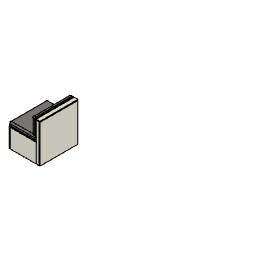
Sofa (Autodesk Fusion 360 design; units mm, degrees)
Autodesk Fusion 360 part; units mm, degrees
sketch "Sketch1" plane through (0, -793.733, 0) normal (0, 1, 0) x (-1, 0, 0)
  line L0 (-1715, -1034) -> (-1715, 1034)
  line L1 (-2315, 1034) -> (-2815, 1034)
  line L2 (-2815, 334) -> (-2315, 334)
  line L3 (-2315, 334) -> (-2315, 1034)
  line L4 (-2315, 1034) -> (-2815, 334) construction
  line L5 (-2815, 1034) -> (-2315, 334) construction
  line L6 (-4545, 1034) -> (-115, 1034)
  line L7 (-2815, 334) -> (-2865, 334)
  line L8 (-2865, 334) -> (-2865, 1034)
  line L9 (-2333, 1016) -> (-2797, 1016)
  line L10 (-2797, 1016) -> (-2797, 352)
  line L11 (-2797, 352) -> (-2333, 352)
  line L12 (-2333, 352) -> (-2333, 1016)
  line L13 (-2333, 1016) -> (-2797, 352) construction
  line L14 (-2797, 1016) -> (-2333, 352) construction
  line L15 (-2865, 334) -> (-2883, 334)
  line L16 (-2883, 334) -> (-2883, 1034)
  line L17 (-2797, 352) -> (-2865, 352)
  line L18 (-2797, 1016) -> (-2865, 1016)
  line L19 (-2815, 1016) -> (-2815, 352)
  line L20 (-2815, 402) -> (-2865, 402)
  line L21 (-2815, 966) -> (-2865, 966)
  line L22 (-2815, 709) -> (-2865, 709)
  line L23 (-2815, 659) -> (-2865, 659)
  line L24 (-2333, 334) -> (-2333, 352)
  line L25 (-2333, 1016) -> (-2333, 1034)
  line L26 (-2815, 1034) -> (-2815, 1016)
  line L27 (-2815, 352) -> (-2815, 334)
  line L28 (-1715, 1034) -> (-3765, 1034)
  line L29 (-3765, 1034) -> (-3765, 0)
  line L30 (-4545, -1034) -> (-1715, -1034)
  line L31 (-3765, 0) -> (-4545, 0)
  line L32 (-4545, 0) -> (-4545, -1034)
  point P0 (-2565, 684)
  point P1 (-2565, 684)
  dimension "d71" = 500
  dimension "d72" = 50
  dimension "d73" = 700
  dimension "d74" = 600
  dimension "d77" = 18
  dimension "d78" = 18
  dimension "d79" = 18
  dimension "d84" = 18
  dimension "d85" = 18
  dimension "d86" = 25
  dimension "d87" = 50
  dimension "d88" = 50
  dimension "d89" = 50
  constraint horizontal L1
  constraint parallel L1 L2
  constraint coincident L4 P1
  constraint coincident L5 P1
  constraint coincident L1.start L6
  constraint horizontal L7
  constraint vertical L8
  constraint coincident L6 L8.end
  constraint horizontal L9
  constraint perpendicular L9 L10
  constraint parallel L9 L11
  constraint parallel L10 L12
  constraint coincident L13 P1
  constraint coincident L14 P1
  constraint coincident P1 P0
  constraint perpendicular L8 L15
  constraint coincident L6 L16.end
  constraint perpendicular L6 L16
  constraint coincident L8 L17.end
  constraint perpendicular L8 L17
  constraint coincident L8 L18.end
  constraint perpendicular L8 L18
  constraint coincident L18 L19.start
  constraint coincident L17 L19.end
  constraint perpendicular L17 L19
  constraint coincident L19 L20.start
  constraint coincident L8 L20.end
  constraint perpendicular L8 L20
  constraint coincident L19 L21.start
  constraint coincident L8 L21.end
  constraint perpendicular L8 L21
  constraint coincident L19 L22.start
  constraint coincident L8 L22.end
  constraint perpendicular L8 L22
  constraint coincident L19 L23.start
  constraint coincident L8 L23.end
  constraint perpendicular L8 L23
  constraint coincident L2 L24.start
  constraint perpendicular L11 L24
  constraint coincident L6 L25.end
  constraint perpendicular L9 L25
  measures "d71" distance of L2.start L2.end
  measures "d72" distance of L2.start L7.end
  measures "d73" distance of L1.start L2.end
  measures "d74" distance of L0 L3
  measures "d77" distance of L3 L12
  measures "d78" distance of L2 L11
  measures "d79" distance of L8 L16
  measures "d84" distance of L10 L19
  measures "d85" distance of L1 L9
  measures "d86" distance of P1 L22
  measures "d87" distance of L22 L23
  measures "d88" distance of L17 L20
  measures "d89" distance of L18 L21
extrude "Extrude1" add sketch "Sketch1" along normal blind 346 contours L1 L2 L3 L6 L12 L24 L25 L28 | L10 L17 L18 L19 makes body 1 at (2315, -678.3997, 567.3333) makes body 2 at (2797, -678.3997, 794.6667)
extrude "Extrude2" add sketch "Sketch1" along normal blind 346 separate body contours L1 L6 L9 L18 L25 L26 L28 | L2 L11 L17 L24 L27 makes body 3 at (2493.6667, -563.0664, 352) makes body 4 at (2493.6667, -563.0664, 1034)
extrude "Extrude3" add sketch "Sketch1" along normal blind 700 separate body contours L6 L8 L18 L26 L28 | L7 L8 L17 L27 makes body 5 at (2831.6667, -327.0664, 334) makes body 6 at (2831.6667, -560.3997, 1016)
extrude "Extrude4" add sketch "Sketch1" along normal blind 700 separate body contours L6 L8 L15 L16 L28 makes body 7
extrude "Extrude1'" add sketch "Sketch1" along normal blind 700 separate body contours L8 L18 L19 L21 | L8 L17 L19 L20 | L8 L19 L22 L23 makes body 8 at (2865, -327.0664, 368.6667) makes body 9 at (2815, -327.0664, 692.3333) makes body 10 at (2815, -327.0664, 999.3333) in component "Wood Support (1)"
extrude "Extrude6" add sketch "Sketch1" along normal blind 18 from surface at 700 separate body contours L6 L8 L18 L26 L28 | L6 L8 L15 L16 L28 | L8 L18 L19 L21 | L7 L8 L17 L27 | L8 L19 L21 L22 | L8 L17 L19 L20 | L8 L19 L22 L23 | L8 L19 L20 L23 makes body 11
extrude "Extrude1''" add sketch "Sketch1" along normal blind 18 from surface at 346 separate body contours L1 L2 L3 L6 L12 L24 L25 L28 | L1 L6 L9 L18 L25 L26 L28 | L9 L10 L11 L12 | L2 L11 L17 L24 L27 | L10 L17 L18 L19 makes body 12 in component "Bottom Pillow"
extrude "Extrude2'" add 1 faces at (2493.6667, -429.733, 692.3333) along direction (0, 1, 0) blind 65 separate body on bodies 12 makes body 13 in component "Bottom Pillow"
extrude "Extrude3'" add 1 faces at (2315, -408.0664, 567.3333) along direction (-1, 0, 0) blind 10 on bodies 13 bodies 13 in component "Bottom Pillow"
extrude "Extrude4'" add 1 faces at (2645, -386.3997, 334) along direction (0, 0, -1) blind 10 on bodies 13 bodies 13 in component "Bottom Pillow"
fillet "Fillet2" radius 25 8 edges at (2305, -397.233, 324) (2815, -397.233, 324) (2560, -364.733, 324) (2815, -364.733, 679) (2815, -397.233, 1034) (2560, -364.733, 1034) (2305, -364.733, 679) (2305, -397.233, 1034) on bodies 13 in component "Bottom Pillow"
fillet "Fillet3" radius 10 8 edges at (2305, -429.733, 679) (2312.3223, -429.733, 1026.6777) (2560, -429.733, 1034) (2807.6777, -429.733, 1026.6777) (2815, -429.733, 679) (2807.6777, -429.733, 331.3223) (2560, -429.733, 324) (2312.3223, -429.733, 331.3223) on bodies 13 in component "Bottom Pillow"
sketch "Sketch1 (2)" plane through (2815, 0, 0) normal (-1, 0, 0) x (0, 0, 1) in component "Back Pillow"
  line L0 (334, -93.733) -> (1034, -93.733)
  line L1 (1034, -93.733) -> (1034, -75.733)
  line L2 (1034, -75.733) -> (334, -75.733)
  line L3 (334, -75.733) -> (334, -93.733)
  line L4 (334, -75.733) -> (1034, -75.733)
  line L5 (1034, -75.733) -> (1034, -369.733)
  line L6 (1034, -369.733) -> (334, -369.733)
  line L7 (334, -369.733) -> (334, -75.733)
  line L8 (1034, 803.733) -> (1034, -803.733)
  line L9 (1009, -389.733) -> (1034, -389.733)
  dimension "d117" = 20
  constraint horizontal L4
  constraint vertical L5
  constraint horizontal L6
  constraint vertical L7
  constraint coincident L2.end L3.start
  constraint coincident L5.end L8
  measures "d117" distance of L5.end L9
extrude "Extrude1'''" add sketch "Sketch1 (2)" along normal blind 18 separate body makes body 14 in component "Back Pillow"
extrude "Extrude2''" add 1 faces at (2797, -277.733, 800.6667) along direction (-1, 0, 0) blind 65 separate body on bodies 14 makes body 15 in component "Back Pillow"
extrude "Extrude3''" add 2 faces at (2753.6667, -81.733, 334) (2775.3333, -277.733, 334) along direction (0, 0, -1) blind 10 on bodies 15 bodies 15 in component "Back Pillow"
extrude "Extrude4''" add 1 faces at (2775.3333, -75.733, 797.3333) along direction (0, 1, 0) blind 10 on bodies 15 bodies 15 in component "Back Pillow"
fillet "Fillet1" radius 25 8 edges at (2732, -217.733, 324) (2732, -65.733, 679) (2764.5, -65.733, 324) (2764.5, -369.733, 324) (2764.5, -369.733, 1034) (2732, -369.733, 679) (2732, -217.733, 1034) (2764.5, -65.733, 1034) on bodies 15 in component "Back Pillow"
fillet "Fillet2'" radius 10 8 edges at (2797, -73.0554, 331.3223) (2797, -65.733, 679) (2797, -73.0554, 1026.6777) (2797, -217.733, 1034) (2797, -362.4107, 1026.6777) (2797, -369.733, 679) (2797, -362.4107, 331.3223) (2797, -217.733, 324) on bodies 15 in component "Back Pillow"
component "Wood Support (1)" placed x (1, 0, 0) y (0, 1, 0) z (0, 0, 1) at (0, 0, 0)
component "Bottom Pillow" placed x (1, 0, 0) y (0, 1, 0) z (0, 0, 1) at (0, 0, 0)
component "Back Pillow" placed x (1, 0, 0) y (0, 1, 0) z (0, 0, 1) at (0, 0, 0)
named bodies: "Front Wall", "Right Wall", "Left Wall", "Middle Wall", "Right Back", "Back Wall"
